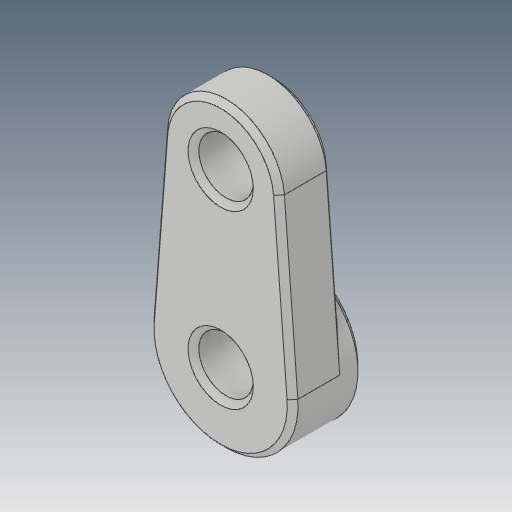
# Autodesk Inventor part: hinge_guid_c
Saved by Autodesk Inventor 2018 (Build 220112000, 112)
## iProperties
Created: 2019-01-31
Part Number: hinge_guid_c
Material: Generic
Document SubType Name: Modeling
Designer: Tsche
Density: 1 g/cm^3
Appearance: Default
Author: Tsche
Autodesk Inventor part; units mm, degrees
ref_plane "YZ Plane" through (0, 0, 0) normal (1, 0, 0) x (0, 1, 0)
ref_plane "XZ Plane" through (0, 0, 0) normal (0, 1, 0) x (-1, 0, 0)
ref_plane "XY Plane" through (0, 0, 0) normal (0, 0, 1) x (1, 0, 0)
sketch "Sketch1" plane through (0, 0, 0) normal (0, 0, 1) x (1, 0, 0)
  circle A0 centre (0, 0) radius 1.5125
  circle A1 centre (0, 9.525) radius 1.5125
  line L0 (0, 0) -> (0, 9.525) construction
  arc A2 (-3.987581, 0.314961) -> (3.987581, 0.314961) centre (0, 0) ccw
  arc A3 (3.239909, 9.780906) -> (-3.239909, 9.780906) centre (0, 9.525) ccw
  line L1 (-3.239909, 9.780906) -> (-3.987581, 0.314961)
  line L2 (3.987581, 0.314961) -> (3.239909, 9.780906)
  dimension "d2" = 9.525
  dimension "d3" = 4
  dimension "d4" = 3.025
  dimension "d7" = 3.25
  constraints: 6 end point, 5 point on circle, 4 centre point, 4 tangent, 2 concentric, 1 coincident, 1 equal radius, 1 vertical
  measures "d2" distance of L0.start L0.end
  measures "d3" radius of A2
  measures "d4" diameter of A0
  measures "d7" radius of A3
extrude "Extrusion1" add sketch "Sketch1" along normal mid plane 2.925
sketch "Sketch2" plane through (0, 0, -1.4625) normal (0, 0, -1) x (-1, 0, 0)
  circle A0 centre (0, 0) radius 1.5125
  arc A1 (-3.987581, 0.314961) -> (3.987581, 0.314961) centre (0, 0) ccw construction
  circle A2 centre (0, 0) radius 4
  constraints: 1 centre point, 1 coincident, 1 concentric
extrude "Extrusion2" add sketch "Sketch2" along normal blind 1
chamfer "Chamfer1" distance 0.3 angle 45 13 edges at (-1.5125, 9.525, -1.4625) (-1.5125, 9.525, 1.4625) (0, 12.775, -1.4625) (3.6137, 5.0479, -1.4625) (-3.6137, 5.0479, -1.4625) (-3.6137, 5.0479, 1.4625) (0, -4, 1.4625) (3.6137, 5.0479, 1.4625) (0, 12.775, 1.4625) (0, 4, -1.4625) (4, 0, -2.4625) (-1.5125, 0, 1.4625) (1.5125, 0, -2.4625)
equation "\"d2\" = hinge_guid_length_c"
equation "\"d3\" = 0.5 * finger_thickness"
equation "\"d4\" = bore_clearance"
equation "\"d7\" = 0.5 * bar_diameter"
equation "\"d5\" = hinge_thickness - finger_link_clearence"
equation "\"d10\" = champfer"
equation "\"bore_press\" = 2.925"
equation "\"bore_clearance\" = 3.025"
equation "\"hinge_act_length_ab\" = 11.049"
equation "\"hinge_act_length_bc\" = 16.66875"
equation "\"bar_diameter\" = 6.5"
equation "\"hinge_thickness\" = 3"
equation "\"finger_width\" = 25"
equation "\"finger_thickness\" = 8"
equation "\"finger_part_A_length\" = 42.8625"
equation "\"finger_part_B_length\" = 28.575"
equation "\"finger_link_width\" = 3.5"
equation "\"finger_link_clearence\" = 0.075"
equation "\"tol\" = 0.5 * finger_link_clearence"
equation "\"link_tol\" = 0.254"
equation "\"bar_thickness\" = 4"
equation "\"bar_width\" = 7"
equation "\"hinge_dist_sym_plane\" = 4"
equation "\"hinge_act_length_c\" = 7.62"
equation "\"hinge_act_length_a\" = 21.43125"
equation "\"hinge_guid_length_c\" = 9.525"
equation "\"hinge_guid_length_bc\" = 9.525"
equation "\"hinge_guid_length_ab\" = 17.145"
equation "\"hinge_guid_length_a\" = 17.145"
equation "\"bar_length_bc\" = finger_part_B_length"
equation "\"bar_act_length_ab\" = 40.48125"
equation "\"bar_guid_length_ab\" = 43.275"
equation "\"champfer\" = 0.3"
equation "\"fillet\" = 0.4"
equation "\"dist_finger_BC\" = 56.5"
equation "\"hinge_point\" = 15"
equation "\"gear_diameter\" = 14"
body "Solid1"
